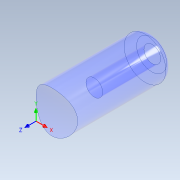
# Autodesk Inventor part: shank
Saved by Autodesk Inventor 2020 (Build 240168000, 168)
## iProperties
Created: 2021-03-27
Part Number: shank
Material: Generic
Document SubType Name: Modeling
Designer: DELL
Density: 1 g/cm^3
Appearance: Clear - Blue
Author: DELL
Autodesk Inventor part; units mm, degrees
ref_plane "YZ Plane" through (0, 0, 0) normal (1, 0, 0) x (0, 1, 0)
ref_plane "XZ Plane" through (0, 0, 0) normal (0, 1, 0) x (-1, 0, 0)
ref_plane "UCS1: YZ Plane" through (0, 0, 0) normal (1, 0, 0) x (0, 1, 0)
sketch "Sketch1" plane through (0, 0, 0) normal (1, 0, 0) x (0, 1, 0)
  circle A0 centre (0, 0) radius 25
  arc A1 (-25, -19.1099) -> (25, -19.1099) centre (0, 31) ccw
  line L0 (0, 31) -> (0, 0) construction
  circle A2 centre (0, 0) radius 140 construction
  line L1 (-25, 0) -> (-25, -140)
  line L2 (-25, -140) -> (25, -140)
  line L3 (25, -140) -> (25, 0)
  line L4 (-25, -140) -> (-40, -140)
  line L5 (-40, -140) -> (-40, -134.1641)
  arc A3 (-40, -134.1641) -> (0, -140) centre (0, 0) ccw
  line L6 (0, 0) -> (0, -140)
  line L7 (-25, 0) -> (25, 0)
  point P0 (0, -25)
  point P1 (-25, -137.7498)
  dimension "d2" = 280
  dimension "d0" = 50
  dimension "d1" = 112
  dimension "d3" = 40
  constraints: 16 end point, 6 point on circle, 4 vertical, 3 centre point, 3 coincident, 3 horizontal, 3 tangent, 2 perpendicular, 2 point on line, 1 midpoint, 3 other
  measures "d0" diameter of A0
  measures "d1" diameter of A1
  measures "d3" distance from line of point (0, 0) L5
sketch "Sketch2" plane through (0, 0, 0) normal (0, 0, 1) x (1, 0, 0)
  circle A0 centre (0, 0) radius 10
  dimension "d7" = 20
  constraints: 1 centre point, 1 coincident
  measures "d7" diameter of A0
revolve "Revolution1" add sketch "Sketch1" angle 360 about axis through (0, 0, 0) along (0, 0, -1) picked at (-1.8543, -16.4577) contours L7 L6 A0 | A0 A1 L1 | L6 A3 L1 A1
extrude "Extrusion1" cut sketch "Sketch1" against normal through all both and the other way through all contours L7 A0 | L3 A1 A0 | A0 L6 L7 | L7 L6 A0 | A0 A1 L1
ref_plane "Work Plane1" through (0, 0, -140) normal (0, 0, 1) x (1, 0, 0)
extrude "Extrusion2" cut sketch "Sketch2" along normal blind 70 from surface at -140
fillet "Fillet1" radius 8 1 edges at (0, 25, -137.7498)
body "Solid1"
